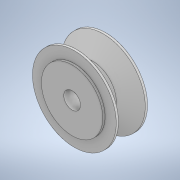
# Autodesk Inventor part: Rand1
Saved by Autodesk Inventor 2022 (Build 260153000, 153)
## iProperties
Created: 2023-06-25
Part Number: Rand1
Material: Generic
Document SubType Name: Modeling
Designer: Eric Cao
Density: 1 g/cm^3
Appearance: Default
Author: Eric Cao
Autodesk Inventor part; units mm, degrees
ref_plane "YZ Plane" through (0, 0, 0) normal (1, 0, 0) x (0, 1, 0)
ref_plane "XZ Plane" through (0, 0, 0) normal (0, 1, 0) x (-1, 0, 0)
ref_plane "XY Plane" through (0, 0, 0) normal (0, 0, 1) x (1, 0, 0)
sketch "Sketch1" plane through (0, 0, 0) normal (1, 0, 0) x (0, 1, 0)
  line L0 (2.9662, 0) -> (2.9662, -32)
  line L1 (2.9662, -32) -> (22.9662, -32)
  line L2 (22.9662, -32) -> (22.9662, -30)
  line L3 (22.9662, -30) -> (32.9662, -30)
  line L4 (32.9662, -30) -> (32.9662, -28)
  line L5 (32.9662, -28) -> (16.5117, -18.5)
  line L6 (16.5117, -18.5) -> (16.5117, -13.5)
  line L7 (16.5117, -13.5) -> (32.9662, -4)
  line L8 (32.9662, -4) -> (32.9662, -2)
  line L9 (32.9662, -2) -> (22.9662, -2)
  line L10 (22.9662, -2) -> (22.9662, 0)
  line L11 (22.9662, 0) -> (2.9662, 0)
  line L12 (0, 0) -> (34.8019, 0) construction
  line L13 (-4.5338, 0.8694) -> (-4.5338, -29.1306)
  dimension "d0" = 32
  dimension "d1" = 20
  dimension "d2" = 2
  dimension "d3" = 10
  dimension "d4" = 2
  dimension "d5" = 5
  dimension "d6" = 2
  dimension "d7" = 10
  dimension "d8" = 2
  dimension "d9" = 60
  dimension "d16" = 32.9662
  dimension "d17" = 1.8357
  dimension "d20" = 30
  dimension "d21" = 15
  constraints: 28 end point, 6 perpendicular, 3 vertical, 2 collinear, 2 point on line, 1 equal length, 1 parallel
  measures "d0" distance of L0.start L0.end
  measures "d1" distance of L0.end L1.end
  measures "d2" distance of L1.end L2.end
  measures "d3" distance of L2.end L3.end
  measures "d4" distance of L3.end L4.end
  measures "d5" distance of L5.end L6.end
  measures "d6" distance of L7.end L8.end
  measures "d7" distance of L8.end L9.end
  measures "d8" distance of L9.end L10.end
  measures "d9" angle of L5 L7
  measures "d16" distance from line of L12.start L4
  measures "d17" distance from line of L12.end L4
  measures "d20" distance of L13.start L13.end
  measures "d21" diameter of L0 L13
revolve "Revolution1" add sketch "Sketch1" angle 360 about axis through (0, -4.5338, 0.8694) along (0, 0, -1)
body "Solid1"
